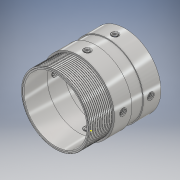
# Autodesk Inventor part: superior
Saved by Autodesk Inventor 2018 (Build 220112000, 112)
## iProperties
Created: 2019-11-08
Part Number: superior
Material: Generic
Document SubType Name: Sheet Metal
Designer: Marie
Density: 1 g/cm^3
Sheet Metal Rule: Default
Appearance: Default
Author: Marie
Autodesk Inventor part; units mm, degrees
ref_plane "XZ Plane" through (0, 0, 0) normal (0, 1, 0) x (-1, 0, 0)
ref_plane "XY Plane" through (0, 0, 0) normal (0, 0, 1) x (1, 0, 0)
sketch "Sketch1" plane through (0, 0, 0) normal (0, 0, 1) x (1, 0, 0)
  line L0 (-1.5, 60) -> (1.5, 60)
  line L1 (1.5, 60) -> (1.5, 45)
  line L2 (1.5, 45) -> (-1.5, 45)
  line L3 (-1.5, 45) -> (-1.5, 60)
  line L4 (-0.75, 45) -> (0.75, 45)
  line L5 (0.75, 45) -> (0.75, 35)
  line L6 (0.75, 35) -> (-0.75, 35)
  line L7 (-0.75, 35) -> (-0.75, 45)
  line L8 (-1.5, 35) -> (1.5, 35)
  line L9 (1.5, 35) -> (1.5, 20)
  line L10 (1.5, 20) -> (-1.5, 20)
  line L11 (-1.5, 20) -> (-1.5, 35)
  line L12 (0, 20) -> (-1.5, 20)
  line L13 (-1.5, 20) -> (-1.5, 0)
  line L14 (-1.5, 0) -> (0, 0)
  line L15 (0, 0) -> (0, 20)
  line L16 (-29.25, 61.1995) -> (-29.25, -4.0597)
  point P0 (0, 0)
  dimension "d1" = 3
  dimension "d2" = 15
  dimension "d4" = 1.5
  dimension "d5" = 10
  dimension "d8" = 3
  dimension "d9" = 15
  dimension "d10" = 1.5
  dimension "d11" = 20
  dimension "d225" = 27.75
  constraints: 34 end point, 8 parallel, 4 horizontal, 4 perpendicular, 1 midpoint, 1 point on line, 1 vertical
  measures "d1" distance of L1.end L2.end
  measures "d2" distance of L0.end L1.end
  measures "d4" distance of L5.end L6.end
  measures "d5" distance of L4.end L5.end
  measures "d8" distance of L9.end L10.end
  measures "d9" distance of L8.end L9.end
  measures "d10" distance of L14.end L13.end
  measures "d11" distance of L13.end L12.end
  measures "d225" distance between parallel lines of L13 L16
revolve "Revolution1" add sketch "Sketch1" angle 360 about axis through (-29.25, 61.1995, 0) along (0, -1, 0)
ref_plane "Work Plane2" through (1.5, 27.5, 0) normal (1, 0, 0) x (0, 1, 0)
sketch "Sketch9" plane through (1.5, 27.5, 0) normal (1, 0, 0) x (0, 1, 0)
  point P0 (-27.5, 0)
  point P1 (23.8502, 0)
  point P2 (0, 0)
hole "Hole1" at (1.5, 51.3502, 0) at (1.5, 27.5, 0) direction (-1, 0, 0) diameter 6 end through all
sketch "Sketch10" plane through (1.5, 27.5, 0) normal (1, 0, 0) x (0, 1, 0)
  point P0 (-27.5, 0)
sketch "Sketch31" plane through (-29.25, 0, 0) normal (-1, 0, 0) x (0, 0, 1)
  line L0 (29.25, 0) -> (29.25, 20)
  line L1 (29.25, 20) -> (27.0256, 20)
  line L2 (27.0256, 20) -> (27.0256, 0)
  line L3 (27.0256, 0) -> (29.25, 0)
  line L4 (0, -15.9256) -> (0, 72.6543) projected
  constraints: 8 end point
revolve "Revolution16" cut sketch "Sketch31" angle 360 about axis through (-29.25, 0, 0) along (0, 1, 0)
sketch "Sketch32" plane through (-29.25, 0, 0) normal (-1, 0, 0) x (0, 0, 1)
  line L0 (29.25, 0) -> (29.25, 20)
  line L1 (29.25, 20) -> (27.0256, 20)
  line L2 (27.0256, 20) -> (27.0256, 0)
  line L3 (27.0256, 0) -> (29.25, 0)
  line L4 (0, -15.9256) -> (0, 72.6543) projected
  constraints: 8 end point
revolve "Revolution17" add sketch "Sketch32" angle 360 about axis through (-29.25, 0, 0) along (0, 1, 0) separate body
thread "Thread13" size "M6x1" class "6H" standard "ANSI Metric M Profile" full length
thread "Thread14" size "M6x1" class "6H" standard "ANSI Metric M Profile" full length
thread "Thread15" size "M6x1" class "6H" standard "ANSI Metric M Profile" full length
thread "Thread16" size "M6x1" class "6H" standard "ANSI Metric M Profile" full length
pattern_circular "Circular Pattern2" count 4 over 360 about axis through (-29.25, 10, 0) along (0, -1, 0) of "Hole1" bodies 1
thread "Thread17" size "M6x1" class "6H" standard "ANSI Metric M Profile" full length
thread "Thread18" size "M6x1" class "6H" standard "ANSI Metric M Profile" full length
thread "Thread19" size "M6x1" class "6H" standard "ANSI Metric M Profile" full length
thread "Thread20" size "M6x1" class "6H" standard "ANSI Metric M Profile" full length
sketch "Sketch34" plane through (-56.8374, 51.3502, 0) normal (0, -1, 0) x (0, 0, 1)
  line L0 (3, 0) -> (3, 3.1626)
  line L1 (3, 3.1626) -> (2.2585, 3.1626)
  line L2 (2.2585, 3.1626) -> (2.2585, 0)
  line L3 (2.2585, 0) -> (3, 0)
  line L4 (0, -70.6399) -> (0, 15.4652) projected
  constraints: 8 end point
revolve "Revolution18" add sketch "Sketch34" angle 360 about axis through (-56.8374, 51.3502, 0) along (-1, 0, 0) separate body
sketch "Sketch33" plane through (-56.8374, 51.3502, 3) normal (0, 1, 0) x (-1, 0, 0)
  line L0 (-0.5834, -0.0507) -> (-0.5001, -0.0507) construction
  line L1 (0.0832, -0.6911) -> (-0.0001, -0.8511) construction
  line L2 (-1.0001, -0.8511) -> (-1.0834, -0.6911) construction
  line L3 (-0.4168, -0.0507) -> (-0.5001, 0.1093) construction
  line L4 (-0.5001, 0.1093) -> (-0.5834, -0.0507) construction
  line L5 (-1.0001, -0.8511) -> (-0.9168, -0.6911) construction
  line L6 (-0.4168, -0.0507) -> (-0.0834, -0.6911)
  line L7 (-1.0834, -0.6911) -> (-0.9168, -0.6911) construction
  arc A0 (-1.0834, -0.6911) -> (-1.0001, -0.7416) centre (-1.0001, -0.6477) ccw construction
  line L8 (0.0832, -0.6911) -> (-0.0834, -0.6911) construction
  line L9 (-1.0001, -0.8511) -> (-1.0001, -0.6911) construction
  line L10 (-0.0001, -0.8511) -> (-0.0001, -0.6911) construction
  line L11 (-0.5001, 0.1093) -> (-0.5001, -0.0002) construction
  line L12 (-1.0001, -0.7416) -> (-0.0001, -0.7416)
  arc A1 (-1.0001, -0.7416) -> (-0.9168, -0.6911) centre (-1.0001, -0.6477) ccw
  line L13 (-0.0834, -0.6911) -> (-0.0001, -0.8511) construction
  line L14 (-0.9168, -0.6911) -> (-0.5834, -0.0507)
  line L15 (-0.0001, -0.0002) -> (-0.0001, 0.0177)
  line L16 (-0.0001, 0.0177) -> (-0.0001, -0.0002)
  line L17 (-0.0001, -0.0002) -> (0.0334, -0.0002)
  arc A2 (-0.0834, -0.6911) -> (-0.0001, -0.7416) centre (-0.0001, -0.6477) ccw
  arc A3 (-0.0001, -0.7416) -> (0.0832, -0.6911) centre (-0.0001, -0.6477) ccw construction
  arc A4 (-0.5001, -0.0002) -> (-0.5834, -0.0507) centre (-0.5001, -0.0941) ccw
  arc A5 (-0.4168, -0.0507) -> (-0.5001, -0.0002) centre (-0.5001, -0.0941) ccw
  line L18 (-0.5001, -0.0002) -> (-0.5001, -0.0507) construction
  line L19 (-0.5001, -0.0507) -> (-0.4168, -0.0507) construction
  dimension "d289" = 55
  dimension "d290" = 0.1601
  dimension "d291" = 0.1601
  dimension "Sketch33_ThreadOffset" = 0
  dimension "Sketch33_MajorRadius" = 0.7415
  dimension "d294" = 1
  dimension "Sketch33_MinorRadius" = 0
  constraints: 40 end point, 12 point on circle, 10 parallel, 8 tangent, 6 centre point, 6 collinear, 2 midpoint, 2 point on line, 1 horizontal, 1 perpendicular, 3 other
  measures "d289" angle of L6 L14
  measures "d290" distance of L3.end L0.end
  measures "d291" distance of L1.end L10.end
  measures "Sketch33_ThreadOffset" distance between parallel lines of L15 L10
  measures "Sketch33_MajorRadius" distance from line of L12 L15.start
  measures "d294" distance from line of L1.end L9
  measures "Sketch33_MinorRadius" distance edge to line of A5 L17
coil "Coil13" sketch "Sketch33" operation cut axis through (-56.8374, 51.3502, 0) along (-1, 0, 0) pitch 1.001 turns 5.157481 hand right bodies 3
sketch "Sketch36" plane through (-56.8374, 27.5, 0) normal (0, -1, 0) x (0, 0, 1)
  line L0 (3, 0) -> (3, 3.1626)
  line L1 (3, 3.1626) -> (2.2585, 3.1626)
  line L2 (2.2585, 3.1626) -> (2.2585, 0)
  line L3 (2.2585, 0) -> (3, 0)
  line L4 (0, -70.7062) -> (0, 15.863) projected
  constraints: 8 end point
revolve "Revolution19" add sketch "Sketch36" angle 360 about axis through (-56.8374, 27.5, 0) along (-1, 0, 0) separate body
sketch "Sketch35" plane through (-56.8374, 27.5, 3) normal (0, 1, 0) x (-1, 0, 0)
  line L0 (-0.5834, -0.0507) -> (-0.5001, -0.0507) construction
  line L1 (0.0832, -0.6911) -> (-0.0001, -0.8511) construction
  line L2 (-1.0001, -0.8511) -> (-1.0834, -0.6911) construction
  line L3 (-0.4168, -0.0507) -> (-0.5001, 0.1093) construction
  line L4 (-0.5001, 0.1093) -> (-0.5834, -0.0507) construction
  line L5 (-1.0001, -0.8511) -> (-0.9168, -0.6911) construction
  line L6 (-0.4168, -0.0507) -> (-0.0834, -0.6911)
  line L7 (-1.0834, -0.6911) -> (-0.9168, -0.6911) construction
  arc A0 (-1.0834, -0.6911) -> (-1.0001, -0.7416) centre (-1.0001, -0.6477) ccw construction
  line L8 (0.0832, -0.6911) -> (-0.0834, -0.6911) construction
  line L9 (-1.0001, -0.8511) -> (-1.0001, -0.6911) construction
  line L10 (-0.0001, -0.8511) -> (-0.0001, -0.6911) construction
  line L11 (-0.5001, 0.1093) -> (-0.5001, -0.0002) construction
  line L12 (-1.0001, -0.7416) -> (-0.0001, -0.7416)
  arc A1 (-1.0001, -0.7416) -> (-0.9168, -0.6911) centre (-1.0001, -0.6477) ccw
  line L13 (-0.0834, -0.6911) -> (-0.0001, -0.8511) construction
  line L14 (-0.9168, -0.6911) -> (-0.5834, -0.0507)
  line L15 (-0.0001, -0.0002) -> (-0.0001, 0.0177)
  line L16 (-0.0001, 0.0177) -> (-0.0001, -0.0002)
  line L17 (-0.0001, -0.0002) -> (0.0334, -0.0002)
  arc A2 (-0.0834, -0.6911) -> (-0.0001, -0.7416) centre (-0.0001, -0.6477) ccw
  arc A3 (-0.0001, -0.7416) -> (0.0832, -0.6911) centre (-0.0001, -0.6477) ccw construction
  arc A4 (-0.5001, -0.0002) -> (-0.5834, -0.0507) centre (-0.5001, -0.0941) ccw
  arc A5 (-0.4168, -0.0507) -> (-0.5001, -0.0002) centre (-0.5001, -0.0941) ccw
  line L18 (-0.5001, -0.0002) -> (-0.5001, -0.0507) construction
  line L19 (-0.5001, -0.0507) -> (-0.4168, -0.0507) construction
  dimension "d307" = 55
  dimension "d308" = 0.1601
  dimension "d309" = 0.1601
  dimension "Sketch35_ThreadOffset" = 0
  dimension "Sketch35_MajorRadius" = 0.7415
  dimension "d312" = 1
  dimension "Sketch35_MinorRadius" = 0
  constraints: 40 end point, 12 point on circle, 10 parallel, 8 tangent, 6 centre point, 6 collinear, 2 midpoint, 2 point on line, 1 horizontal, 1 perpendicular, 3 other
  measures "d307" angle of L6 L14
  measures "d308" distance of L3.end L0.end
  measures "d309" distance of L1.end L10.end
  measures "Sketch35_ThreadOffset" distance between parallel lines of L15 L10
  measures "Sketch35_MajorRadius" distance from line of L12 L15.start
  measures "d312" distance from line of L1.end L9
  measures "Sketch35_MinorRadius" distance edge to line of A5 L17
coil "Coil14" sketch "Sketch35" operation cut axis through (-56.8374, 27.5, 0) along (-1, 0, 0) pitch 1.001 turns 5.157481 hand right bodies 4
sketch "Sketch38" plane through (1.5, 51.3502, 0) normal (0, -1, 0) x (0, 0, 1)
  line L0 (3, 0) -> (3, 3.1626)
  line L1 (3, 3.1626) -> (2.2585, 3.1626)
  line L2 (2.2585, 3.1626) -> (2.2585, 0)
  line L3 (2.2585, 0) -> (3, 0)
  line L4 (0, -13.6753) -> (0, 74.4181) projected
  constraints: 8 end point
revolve "Revolution20" add sketch "Sketch38" angle 360 about axis through (1.5, 51.3502, 0) along (-1, 0, 0) separate body
sketch "Sketch37" plane through (1.5, 51.3502, 3) normal (0, 1, 0) x (-1, 0, 0)
  line L0 (-0.5834, -0.0507) -> (-0.5001, -0.0507) construction
  line L1 (0.0832, -0.6911) -> (-0.0001, -0.8511) construction
  line L2 (-1.0001, -0.8511) -> (-1.0834, -0.6911) construction
  line L3 (-0.4168, -0.0507) -> (-0.5001, 0.1093) construction
  line L4 (-0.5001, 0.1093) -> (-0.5834, -0.0507) construction
  line L5 (-1.0001, -0.8511) -> (-0.9168, -0.6911) construction
  line L6 (-0.4168, -0.0507) -> (-0.0834, -0.6911)
  line L7 (-1.0834, -0.6911) -> (-0.9168, -0.6911) construction
  arc A0 (-1.0834, -0.6911) -> (-1.0001, -0.7416) centre (-1.0001, -0.6477) ccw construction
  line L8 (0.0832, -0.6911) -> (-0.0834, -0.6911) construction
  line L9 (-1.0001, -0.8511) -> (-1.0001, -0.6911) construction
  line L10 (-0.0001, -0.8511) -> (-0.0001, -0.6911) construction
  line L11 (-0.5001, 0.1093) -> (-0.5001, -0.0002) construction
  line L12 (-1.0001, -0.7416) -> (-0.0001, -0.7416)
  arc A1 (-1.0001, -0.7416) -> (-0.9168, -0.6911) centre (-1.0001, -0.6477) ccw
  line L13 (-0.0834, -0.6911) -> (-0.0001, -0.8511) construction
  line L14 (-0.9168, -0.6911) -> (-0.5834, -0.0507)
  line L15 (-0.0001, -0.0002) -> (-0.0001, 0.0177)
  line L16 (-0.0001, 0.0177) -> (-0.0001, -0.0002)
  line L17 (-0.0001, -0.0002) -> (0.0334, -0.0002)
  arc A2 (-0.0834, -0.6911) -> (-0.0001, -0.7416) centre (-0.0001, -0.6477) ccw
  arc A3 (-0.0001, -0.7416) -> (0.0832, -0.6911) centre (-0.0001, -0.6477) ccw construction
  arc A4 (-0.5001, -0.0002) -> (-0.5834, -0.0507) centre (-0.5001, -0.0941) ccw
  arc A5 (-0.4168, -0.0507) -> (-0.5001, -0.0002) centre (-0.5001, -0.0941) ccw
  line L18 (-0.5001, -0.0002) -> (-0.5001, -0.0507) construction
  line L19 (-0.5001, -0.0507) -> (-0.4168, -0.0507) construction
  dimension "d325" = 55
  dimension "d326" = 0.1601
  dimension "d327" = 0.1601
  dimension "Sketch37_ThreadOffset" = 0
  dimension "Sketch37_MajorRadius" = 0.7415
  dimension "d330" = 1
  dimension "Sketch37_MinorRadius" = 0
  constraints: 40 end point, 12 point on circle, 10 parallel, 8 tangent, 6 centre point, 6 collinear, 2 midpoint, 2 point on line, 1 horizontal, 1 perpendicular, 3 other
  measures "d325" angle of L6 L14
  measures "d326" distance of L3.end L0.end
  measures "d327" distance of L1.end L10.end
  measures "Sketch37_ThreadOffset" distance between parallel lines of L15 L10
  measures "Sketch37_MajorRadius" distance from line of L12 L15.start
  measures "d330" distance from line of L1.end L9
  measures "Sketch37_MinorRadius" distance edge to line of A5 L17
coil "Coil15" sketch "Sketch37" operation cut axis through (1.5, 51.3502, 0) along (-1, 0, 0) pitch 1.001 turns 5.157481 hand right bodies 5
sketch "Sketch40" plane through (1.5, 27.5, 0) normal (0, -1, 0) x (0, 0, 1)
  line L0 (3, 0) -> (3, 3.1626)
  line L1 (3, 3.1626) -> (2.2585, 3.1626)
  line L2 (2.2585, 3.1626) -> (2.2585, 0)
  line L3 (2.2585, 0) -> (3, 0)
  line L4 (0, -13.6753) -> (0, 74.4181) projected
  constraints: 8 end point
revolve "Revolution21" add sketch "Sketch40" angle 360 about axis through (1.5, 27.5, 0) along (-1, 0, 0) separate body
sketch "Sketch39" plane through (1.5, 27.5, 3) normal (0, 1, 0) x (-1, 0, 0)
  line L0 (-0.5834, -0.0507) -> (-0.5001, -0.0507) construction
  line L1 (0.0832, -0.6911) -> (-0.0001, -0.8511) construction
  line L2 (-1.0001, -0.8511) -> (-1.0834, -0.6911) construction
  line L3 (-0.4168, -0.0507) -> (-0.5001, 0.1093) construction
  line L4 (-0.5001, 0.1093) -> (-0.5834, -0.0507) construction
  line L5 (-1.0001, -0.8511) -> (-0.9168, -0.6911) construction
  line L6 (-0.4168, -0.0507) -> (-0.0834, -0.6911)
  line L7 (-1.0834, -0.6911) -> (-0.9168, -0.6911) construction
  arc A0 (-1.0834, -0.6911) -> (-1.0001, -0.7416) centre (-1.0001, -0.6477) ccw construction
  line L8 (0.0832, -0.6911) -> (-0.0834, -0.6911) construction
  line L9 (-1.0001, -0.8511) -> (-1.0001, -0.6911) construction
  line L10 (-0.0001, -0.8511) -> (-0.0001, -0.6911) construction
  line L11 (-0.5001, 0.1093) -> (-0.5001, -0.0002) construction
  line L12 (-1.0001, -0.7416) -> (-0.0001, -0.7416)
  arc A1 (-1.0001, -0.7416) -> (-0.9168, -0.6911) centre (-1.0001, -0.6477) ccw
  line L13 (-0.0834, -0.6911) -> (-0.0001, -0.8511) construction
  line L14 (-0.9168, -0.6911) -> (-0.5834, -0.0507)
  line L15 (-0.0001, -0.0002) -> (-0.0001, 0.0177)
  line L16 (-0.0001, 0.0177) -> (-0.0001, -0.0002)
  line L17 (-0.0001, -0.0002) -> (0.0334, -0.0002)
  arc A2 (-0.0834, -0.6911) -> (-0.0001, -0.7416) centre (-0.0001, -0.6477) ccw
  arc A3 (-0.0001, -0.7416) -> (0.0832, -0.6911) centre (-0.0001, -0.6477) ccw construction
  arc A4 (-0.5001, -0.0002) -> (-0.5834, -0.0507) centre (-0.5001, -0.0941) ccw
  arc A5 (-0.4168, -0.0507) -> (-0.5001, -0.0002) centre (-0.5001, -0.0941) ccw
  line L18 (-0.5001, -0.0002) -> (-0.5001, -0.0507) construction
  line L19 (-0.5001, -0.0507) -> (-0.4168, -0.0507) construction
  dimension "d343" = 55
  dimension "d344" = 0.1601
  dimension "d345" = 0.1601
  dimension "Sketch39_ThreadOffset" = 0
  dimension "Sketch39_MajorRadius" = 0.7415
  dimension "d348" = 1
  dimension "Sketch39_MinorRadius" = 0
  constraints: 40 end point, 12 point on circle, 10 parallel, 8 tangent, 6 centre point, 6 collinear, 2 midpoint, 2 point on line, 1 horizontal, 1 perpendicular, 3 other
  measures "d343" angle of L6 L14
  measures "d344" distance of L3.end L0.end
  measures "d345" distance of L1.end L10.end
  measures "Sketch39_ThreadOffset" distance between parallel lines of L15 L10
  measures "Sketch39_MajorRadius" distance from line of L12 L15.start
  measures "d348" distance from line of L1.end L9
  measures "Sketch39_MinorRadius" distance edge to line of A5 L17
coil "Coil16" sketch "Sketch39" operation cut axis through (1.5, 27.5, 0) along (-1, 0, 0) pitch 1.001 turns 5.157481 hand right bodies 6
sketch "Sketch42" plane through (-29.25, 51.3502, -27.5874) normal (-1, 0, 0) x (0, 1, 0)
  line L0 (3, 0) -> (3, 3.1626)
  line L1 (3, 3.1626) -> (2.2585, 3.1626)
  line L2 (2.2585, 3.1626) -> (2.2585, 0)
  line L3 (2.2585, 0) -> (3, 0)
  line L4 (0, -70.6399) -> (0, 15.4652) projected
  constraints: 8 end point
revolve "Revolution22" add sketch "Sketch42" angle 360 about axis through (-29.25, 51.3502, -27.5874) along (0, 0, -1) separate body
sketch "Sketch41" plane through (-29.25, 54.3502, -27.5874) normal (1, 0, 0) x (0, 0, -1)
  line L0 (-0.5834, -0.0507) -> (-0.5001, -0.0507) construction
  line L1 (0.0832, -0.6911) -> (-0.0001, -0.8511) construction
  line L2 (-1.0001, -0.8511) -> (-1.0834, -0.6911) construction
  line L3 (-0.4168, -0.0507) -> (-0.5001, 0.1093) construction
  line L4 (-0.5001, 0.1093) -> (-0.5834, -0.0507) construction
  line L5 (-1.0001, -0.8511) -> (-0.9168, -0.6911) construction
  line L6 (-0.4168, -0.0507) -> (-0.0834, -0.6911)
  line L7 (-1.0834, -0.6911) -> (-0.9168, -0.6911) construction
  arc A0 (-1.0834, -0.6911) -> (-1.0001, -0.7416) centre (-1.0001, -0.6477) ccw construction
  line L8 (0.0832, -0.6911) -> (-0.0834, -0.6911) construction
  line L9 (-1.0001, -0.8511) -> (-1.0001, -0.6911) construction
  line L10 (-0.0001, -0.8511) -> (-0.0001, -0.6911) construction
  line L11 (-0.5001, 0.1093) -> (-0.5001, -0.0002) construction
  line L12 (-1.0001, -0.7416) -> (-0.0001, -0.7416)
  arc A1 (-1.0001, -0.7416) -> (-0.9168, -0.6911) centre (-1.0001, -0.6477) ccw
  line L13 (-0.0834, -0.6911) -> (-0.0001, -0.8511) construction
  line L14 (-0.9168, -0.6911) -> (-0.5834, -0.0507)
  line L15 (-0.0001, -0.0002) -> (-0.0001, 0.0177)
  line L16 (-0.0001, 0.0177) -> (-0.0001, -0.0002)
  line L17 (-0.0001, -0.0002) -> (0.0334, -0.0002)
  arc A2 (-0.0834, -0.6911) -> (-0.0001, -0.7416) centre (-0.0001, -0.6477) ccw
  arc A3 (-0.0001, -0.7416) -> (0.0832, -0.6911) centre (-0.0001, -0.6477) ccw construction
  arc A4 (-0.5001, -0.0002) -> (-0.5834, -0.0507) centre (-0.5001, -0.0941) ccw
  arc A5 (-0.4168, -0.0507) -> (-0.5001, -0.0002) centre (-0.5001, -0.0941) ccw
  line L18 (-0.5001, -0.0002) -> (-0.5001, -0.0507) construction
  line L19 (-0.5001, -0.0507) -> (-0.4168, -0.0507) construction
  dimension "d361" = 55
  dimension "d362" = 0.1601
  dimension "d363" = 0.1601
  dimension "Sketch41_ThreadOffset" = 0
  dimension "Sketch41_MajorRadius" = 0.7415
  dimension "d366" = 1
  dimension "Sketch41_MinorRadius" = 0
  constraints: 40 end point, 12 point on circle, 10 parallel, 8 tangent, 6 centre point, 6 collinear, 2 midpoint, 2 point on line, 1 horizontal, 1 perpendicular, 3 other
  measures "d361" angle of L6 L14
  measures "d362" distance of L3.end L0.end
  measures "d363" distance of L1.end L10.end
  measures "Sketch41_ThreadOffset" distance between parallel lines of L15 L10
  measures "Sketch41_MajorRadius" distance from line of L12 L15.start
  measures "d366" distance from line of L1.end L9
  measures "Sketch41_MinorRadius" distance edge to line of A5 L17
coil "Coil17" sketch "Sketch41" operation cut axis through (-29.25, 51.3502, -27.5874) along (0, 0, -1) pitch 1.001 turns 5.157481 hand right bodies 7
sketch "Sketch44" plane through (-29.25, 27.5, -27.5874) normal (-1, 0, 0) x (0, 1, 0)
  line L0 (3, 0) -> (3, 3.1626)
  line L1 (3, 3.1626) -> (2.2585, 3.1626)
  line L2 (2.2585, 3.1626) -> (2.2585, 0)
  line L3 (2.2585, 0) -> (3, 0)
  line L4 (0, -70.7062) -> (0, 15.863) projected
  constraints: 8 end point
revolve "Revolution23" add sketch "Sketch44" angle 360 about axis through (-29.25, 27.5, -27.5874) along (0, 0, -1) separate body
sketch "Sketch43" plane through (-29.25, 30.5, -27.5874) normal (1, 0, 0) x (0, 0, -1)
  line L0 (-0.5834, -0.0507) -> (-0.5001, -0.0507) construction
  line L1 (0.0832, -0.6911) -> (-0.0001, -0.8511) construction
  line L2 (-1.0001, -0.8511) -> (-1.0834, -0.6911) construction
  line L3 (-0.4168, -0.0507) -> (-0.5001, 0.1093) construction
  line L4 (-0.5001, 0.1093) -> (-0.5834, -0.0507) construction
  line L5 (-1.0001, -0.8511) -> (-0.9168, -0.6911) construction
  line L6 (-0.4168, -0.0507) -> (-0.0834, -0.6911)
  line L7 (-1.0834, -0.6911) -> (-0.9168, -0.6911) construction
  arc A0 (-1.0834, -0.6911) -> (-1.0001, -0.7416) centre (-1.0001, -0.6477) ccw construction
  line L8 (0.0832, -0.6911) -> (-0.0834, -0.6911) construction
  line L9 (-1.0001, -0.8511) -> (-1.0001, -0.6911) construction
  line L10 (-0.0001, -0.8511) -> (-0.0001, -0.6911) construction
  line L11 (-0.5001, 0.1093) -> (-0.5001, -0.0002) construction
  line L12 (-1.0001, -0.7416) -> (-0.0001, -0.7416)
  arc A1 (-1.0001, -0.7416) -> (-0.9168, -0.6911) centre (-1.0001, -0.6477) ccw
  line L13 (-0.0834, -0.6911) -> (-0.0001, -0.8511) construction
  line L14 (-0.9168, -0.6911) -> (-0.5834, -0.0507)
  line L15 (-0.0001, -0.0002) -> (-0.0001, 0.0177)
  line L16 (-0.0001, 0.0177) -> (-0.0001, -0.0002)
  line L17 (-0.0001, -0.0002) -> (0.0334, -0.0002)
  arc A2 (-0.0834, -0.6911) -> (-0.0001, -0.7416) centre (-0.0001, -0.6477) ccw
  arc A3 (-0.0001, -0.7416) -> (0.0832, -0.6911) centre (-0.0001, -0.6477) ccw construction
  arc A4 (-0.5001, -0.0002) -> (-0.5834, -0.0507) centre (-0.5001, -0.0941) ccw
  arc A5 (-0.4168, -0.0507) -> (-0.5001, -0.0002) centre (-0.5001, -0.0941) ccw
  line L18 (-0.5001, -0.0002) -> (-0.5001, -0.0507) construction
  line L19 (-0.5001, -0.0507) -> (-0.4168, -0.0507) construction
  dimension "d379" = 55
  dimension "d380" = 0.1601
  dimension "d381" = 0.1601
  dimension "Sketch43_ThreadOffset" = 0
  dimension "Sketch43_MajorRadius" = 0.7415
  dimension "d384" = 1
  dimension "Sketch43_MinorRadius" = 0
  constraints: 40 end point, 12 point on circle, 10 parallel, 8 tangent, 6 centre point, 6 collinear, 2 midpoint, 2 point on line, 1 horizontal, 1 perpendicular, 3 other
  measures "d379" angle of L6 L14
  measures "d380" distance of L3.end L0.end
  measures "d381" distance of L1.end L10.end
  measures "Sketch43_ThreadOffset" distance between parallel lines of L15 L10
  measures "Sketch43_MajorRadius" distance from line of L12 L15.start
  measures "d384" distance from line of L1.end L9
  measures "Sketch43_MinorRadius" distance edge to line of A5 L17
coil "Coil18" sketch "Sketch43" operation cut axis through (-29.25, 27.5, -27.5874) along (0, 0, -1) pitch 1.001 turns 5.157481 hand right bodies 8
sketch "Sketch46" plane through (-29.25, 51.3502, 30.75) normal (-1, 0, 0) x (0, 1, 0)
  line L0 (3, 0) -> (3, 3.1626)
  line L1 (3, 3.1626) -> (2.2585, 3.1626)
  line L2 (2.2585, 3.1626) -> (2.2585, 0)
  line L3 (2.2585, 0) -> (3, 0)
  line L4 (0, -13.6753) -> (0, 74.4181) projected
  constraints: 8 end point
revolve "Revolution24" add sketch "Sketch46" angle 360 about axis through (-29.25, 51.3502, 30.75) along (0, 0, -1) separate body
sketch "Sketch45" plane through (-29.25, 54.3502, 30.75) normal (1, 0, 0) x (0, 0, -1)
  line L0 (-0.5834, -0.0507) -> (-0.5001, -0.0507) construction
  line L1 (0.0832, -0.6911) -> (-0.0001, -0.8511) construction
  line L2 (-1.0001, -0.8511) -> (-1.0834, -0.6911) construction
  line L3 (-0.4168, -0.0507) -> (-0.5001, 0.1093) construction
  line L4 (-0.5001, 0.1093) -> (-0.5834, -0.0507) construction
  line L5 (-1.0001, -0.8511) -> (-0.9168, -0.6911) construction
  line L6 (-0.4168, -0.0507) -> (-0.0834, -0.6911)
  line L7 (-1.0834, -0.6911) -> (-0.9168, -0.6911) construction
  arc A0 (-1.0834, -0.6911) -> (-1.0001, -0.7416) centre (-1.0001, -0.6477) ccw construction
  line L8 (0.0832, -0.6911) -> (-0.0834, -0.6911) construction
  line L9 (-1.0001, -0.8511) -> (-1.0001, -0.6911) construction
  line L10 (-0.0001, -0.8511) -> (-0.0001, -0.6911) construction
  line L11 (-0.5001, 0.1093) -> (-0.5001, -0.0002) construction
  line L12 (-1.0001, -0.7416) -> (-0.0001, -0.7416)
  arc A1 (-1.0001, -0.7416) -> (-0.9168, -0.6911) centre (-1.0001, -0.6477) ccw
  line L13 (-0.0834, -0.6911) -> (-0.0001, -0.8511) construction
  line L14 (-0.9168, -0.6911) -> (-0.5834, -0.0507)
  line L15 (-0.0001, -0.0002) -> (-0.0001, 0.0177)
  line L16 (-0.0001, 0.0177) -> (-0.0001, -0.0002)
  line L17 (-0.0001, -0.0002) -> (0.0334, -0.0002)
  arc A2 (-0.0834, -0.6911) -> (-0.0001, -0.7416) centre (-0.0001, -0.6477) ccw
  arc A3 (-0.0001, -0.7416) -> (0.0832, -0.6911) centre (-0.0001, -0.6477) ccw construction
  arc A4 (-0.5001, -0.0002) -> (-0.5834, -0.0507) centre (-0.5001, -0.0941) ccw
  arc A5 (-0.4168, -0.0507) -> (-0.5001, -0.0002) centre (-0.5001, -0.0941) ccw
  line L18 (-0.5001, -0.0002) -> (-0.5001, -0.0507) construction
  line L19 (-0.5001, -0.0507) -> (-0.4168, -0.0507) construction
  dimension "d397" = 55
  dimension "d398" = 0.1601
  dimension "d399" = 0.1601
  dimension "Sketch45_ThreadOffset" = 0
  dimension "Sketch45_MajorRadius" = 0.7415
  dimension "d402" = 1
  dimension "Sketch45_MinorRadius" = 0
  constraints: 40 end point, 12 point on circle, 10 parallel, 8 tangent, 6 centre point, 6 collinear, 2 midpoint, 2 point on line, 1 horizontal, 1 perpendicular, 3 other
  measures "d397" angle of L6 L14
  measures "d398" distance of L3.end L0.end
  measures "d399" distance of L1.end L10.end
  measures "Sketch45_ThreadOffset" distance between parallel lines of L15 L10
  measures "Sketch45_MajorRadius" distance from line of L12 L15.start
  measures "d402" distance from line of L1.end L9
  measures "Sketch45_MinorRadius" distance edge to line of A5 L17
coil "Coil19" sketch "Sketch45" operation cut axis through (-29.25, 51.3502, 30.75) along (0, 0, -1) pitch 1.001 turns 5.157481 hand right bodies 9
sketch "Sketch48" plane through (-29.25, 27.5, 30.75) normal (-1, 0, 0) x (0, 1, 0)
  line L0 (3, 0) -> (3, 3.1626)
  line L1 (3, 3.1626) -> (2.2585, 3.1626)
  line L2 (2.2585, 3.1626) -> (2.2585, 0)
  line L3 (2.2585, 0) -> (3, 0)
  line L4 (0, -13.6753) -> (0, 74.4181) projected
  constraints: 8 end point
revolve "Revolution25" add sketch "Sketch48" angle 360 about axis through (-29.25, 27.5, 30.75) along (0, 0, -1) separate body
sketch "Sketch47" plane through (-29.25, 30.5, 30.75) normal (1, 0, 0) x (0, 0, -1)
  line L0 (-0.5834, -0.0507) -> (-0.5001, -0.0507) construction
  line L1 (0.0832, -0.6911) -> (-0.0001, -0.8511) construction
  line L2 (-1.0001, -0.8511) -> (-1.0834, -0.6911) construction
  line L3 (-0.4168, -0.0507) -> (-0.5001, 0.1093) construction
  line L4 (-0.5001, 0.1093) -> (-0.5834, -0.0507) construction
  line L5 (-1.0001, -0.8511) -> (-0.9168, -0.6911) construction
  line L6 (-0.4168, -0.0507) -> (-0.0834, -0.6911)
  line L7 (-1.0834, -0.6911) -> (-0.9168, -0.6911) construction
  arc A0 (-1.0834, -0.6911) -> (-1.0001, -0.7416) centre (-1.0001, -0.6477) ccw construction
  line L8 (0.0832, -0.6911) -> (-0.0834, -0.6911) construction
  line L9 (-1.0001, -0.8511) -> (-1.0001, -0.6911) construction
  line L10 (-0.0001, -0.8511) -> (-0.0001, -0.6911) construction
  line L11 (-0.5001, 0.1093) -> (-0.5001, -0.0002) construction
  line L12 (-1.0001, -0.7416) -> (-0.0001, -0.7416)
  arc A1 (-1.0001, -0.7416) -> (-0.9168, -0.6911) centre (-1.0001, -0.6477) ccw
  line L13 (-0.0834, -0.6911) -> (-0.0001, -0.8511) construction
  line L14 (-0.9168, -0.6911) -> (-0.5834, -0.0507)
  line L15 (-0.0001, -0.0002) -> (-0.0001, 0.0177)
  line L16 (-0.0001, 0.0177) -> (-0.0001, -0.0002)
  line L17 (-0.0001, -0.0002) -> (0.0334, -0.0002)
  arc A2 (-0.0834, -0.6911) -> (-0.0001, -0.7416) centre (-0.0001, -0.6477) ccw
  arc A3 (-0.0001, -0.7416) -> (0.0832, -0.6911) centre (-0.0001, -0.6477) ccw construction
  arc A4 (-0.5001, -0.0002) -> (-0.5834, -0.0507) centre (-0.5001, -0.0941) ccw
  arc A5 (-0.4168, -0.0507) -> (-0.5001, -0.0002) centre (-0.5001, -0.0941) ccw
  line L18 (-0.5001, -0.0002) -> (-0.5001, -0.0507) construction
  line L19 (-0.5001, -0.0507) -> (-0.4168, -0.0507) construction
  dimension "d415" = 55
  dimension "d416" = 0.1601
  dimension "d417" = 0.1601
  dimension "Sketch47_ThreadOffset" = 0
  dimension "Sketch47_MajorRadius" = 0.7415
  dimension "d420" = 1
  dimension "Sketch47_MinorRadius" = 0
  constraints: 40 end point, 12 point on circle, 10 parallel, 8 tangent, 6 centre point, 6 collinear, 2 midpoint, 2 point on line, 1 horizontal, 1 perpendicular, 3 other
  measures "d415" angle of L6 L14
  measures "d416" distance of L3.end L0.end
  measures "d417" distance of L1.end L10.end
  measures "Sketch47_ThreadOffset" distance between parallel lines of L15 L10
  measures "Sketch47_MajorRadius" distance from line of L12 L15.start
  measures "d420" distance from line of L1.end L9
  measures "Sketch47_MinorRadius" distance edge to line of A5 L17
coil "Coil20" sketch "Sketch47" operation cut axis through (-29.25, 27.5, 30.75) along (0, 0, -1) pitch 1.001 turns 5.157481 hand right bodies 10
thread "Thread22" size "M60x1.5" class "6g" standard "ANSI Metric M Profile" full length
sketch "Sketch53" plane through (-29.25, 0, 0) normal (-1, 0, 0) x (0, 0, 1)
  line L0 (29.25, 0) -> (29.25, 20)
  line L1 (29.25, 20) -> (28.1378, 20)
  line L2 (28.1378, 20) -> (28.1378, 0)
  line L3 (28.1378, 0) -> (29.25, 0)
  line L4 (0, -13.9629) -> (0, 72.3271) projected
  constraints: 8 end point
revolve "Revolution28" cut sketch "Sketch53" angle 360 about axis through (-29.25, 0, 0) along (0, 1, 0) bodies 1
sketch "Sketch54" plane through (-29.25, 0, 0) normal (-1, 0, 0) x (0, 0, 1)
  line L0 (29.25, 0) -> (29.25, 20)
  line L1 (29.25, 20) -> (28.1378, 20)
  line L2 (28.1378, 20) -> (28.1378, 0)
  line L3 (28.1378, 0) -> (29.25, 0)
  line L4 (0, -13.9629) -> (0, 72.3271) projected
  constraints: 8 end point
revolve "Revolution29" add sketch "Sketch54" angle 360 about axis through (-29.25, 0, 0) along (0, 1, 0) separate body
sketch "Sketch52" plane through (-29.25, 0, 0) normal (1, 0, 0) x (0, 1, 0)
  line L0 (-0.8751, -28.2138) -> (-0.7501, -28.2138) construction
  line L1 (0.1249, -29.1743) -> (-0.0001, -29.4144) construction
  line L2 (-1.5001, -29.4144) -> (-1.6251, -29.1743) construction
  line L3 (-0.6251, -28.2138) -> (-0.7501, -27.9737) construction
  line L4 (-0.7501, -27.9737) -> (-0.8751, -28.2138) construction
  line L5 (-1.5001, -29.4144) -> (-1.3751, -29.1743) construction
  line L6 (-0.6251, -28.2138) -> (-0.1251, -29.1743)
  line L7 (-1.6251, -29.1743) -> (-1.3751, -29.1743) construction
  arc A0 (-1.6251, -29.1743) -> (-1.5001, -29.2502) centre (-1.5001, -29.1092) ccw construction
  line L8 (0.1249, -29.1743) -> (-0.1251, -29.1743) construction
  line L9 (-1.5001, -29.4144) -> (-1.5001, -29.1743) construction
  line L10 (-0.0001, -29.4144) -> (-0.0001, -29.1743) construction
  line L11 (-0.7501, -27.9737) -> (-0.7501, -28.138) construction
  line L12 (-1.5001, -29.2502) -> (-0.0001, -29.2502)
  arc A1 (-1.5001, -29.2502) -> (-1.3751, -29.1743) centre (-1.5001, -29.1092) ccw
  line L13 (-0.1251, -29.1743) -> (-0.0001, -29.4144) construction
  line L14 (-1.3751, -29.1743) -> (-0.8751, -28.2138)
  line L15 (-0.0001, -0.0002) -> (-0.0001, 0.0177)
  line L16 (-0.0001, 0.0177) -> (-0.0001, -0.0002)
  line L17 (-0.0001, -0.0002) -> (0.0334, -0.0002)
  arc A2 (-0.1251, -29.1743) -> (-0.0001, -29.2502) centre (-0.0001, -29.1092) ccw
  arc A3 (-0.0001, -29.2502) -> (0.1249, -29.1743) centre (-0.0001, -29.1092) ccw construction
  arc A4 (-0.7501, -28.138) -> (-0.8751, -28.2138) centre (-0.7501, -28.2789) ccw
  arc A5 (-0.6251, -28.2138) -> (-0.7501, -28.138) centre (-0.7501, -28.2789) ccw
  line L18 (-0.7501, -28.138) -> (-0.7501, -28.2138) construction
  line L19 (-0.7501, -28.2138) -> (-0.6251, -28.2138) construction
  dimension "d456" = 55
  dimension "d457" = 0.2401
  dimension "d458" = 0.2401
  dimension "Sketch52_ThreadOffset" = 0
  dimension "Sketch52_MajorRadius" = 29.25
  dimension "d461" = 1.5
  dimension "Sketch52_MinorRadius" = 28.1378
  constraints: 40 end point, 12 point on circle, 10 parallel, 8 tangent, 6 centre point, 6 collinear, 2 midpoint, 2 point on line, 1 horizontal, 1 perpendicular, 3 other
  measures "d456" angle of L6 L14
  measures "d457" distance of L3.end L0.end
  measures "d458" distance of L1.end L10.end
  measures "Sketch52_ThreadOffset" distance between parallel lines of L15 L10
  measures "Sketch52_MajorRadius" distance from line of L12 L15.start
  measures "d461" distance from line of L1.end L9
  measures "Sketch52_MinorRadius" distance edge to line of A5 L17
coil "Coil22" sketch "Sketch52" operation cut axis through (-29.25, 0, 0) along (0, 1, 0) pitch 1.5015 turns 15.318015 hand right bodies 11
equation "\"d60\" = Thickness"
equation "\"d289\" = d296"
equation "\"d290\" = 0.160083 * Sketch33_Pitch"
equation "\"d291\" = 0.160083 * Sketch33_Pitch"
equation "\"d294\" = Sketch33_Pitch"
equation "\"d307\" = d314"
equation "\"d308\" = 0.160083 * Sketch35_Pitch"
equation "\"d309\" = 0.160083 * Sketch35_Pitch"
equation "\"d312\" = Sketch35_Pitch"
equation "\"d325\" = d332"
equation "\"d326\" = 0.160083 * Sketch37_Pitch"
equation "\"d327\" = 0.160083 * Sketch37_Pitch"
equation "\"d330\" = Sketch37_Pitch"
equation "\"d343\" = d350"
equation "\"d344\" = 0.160083 * Sketch39_Pitch"
equation "\"d345\" = 0.160083 * Sketch39_Pitch"
equation "\"d348\" = Sketch39_Pitch"
equation "\"d361\" = d368"
equation "\"d362\" = 0.160083 * Sketch41_Pitch"
equation "\"d363\" = 0.160083 * Sketch41_Pitch"
equation "\"d366\" = Sketch41_Pitch"
equation "\"d379\" = d386"
equation "\"d380\" = 0.160083 * Sketch43_Pitch"
equation "\"d381\" = 0.160083 * Sketch43_Pitch"
equation "\"d384\" = Sketch43_Pitch"
equation "\"d397\" = d404"
equation "\"d398\" = 0.160083 * Sketch45_Pitch"
equation "\"d399\" = 0.160083 * Sketch45_Pitch"
equation "\"d402\" = Sketch45_Pitch"
equation "\"d415\" = d422"
equation "\"d416\" = 0.160083 * Sketch47_Pitch"
equation "\"d417\" = 0.160083 * Sketch47_Pitch"
equation "\"d420\" = Sketch47_Pitch"
equation "\"d456\" = d463"
equation "\"d457\" = 0.160083 * Sketch52_Pitch"
equation "\"d458\" = 0.160083 * Sketch52_Pitch"
equation "\"d461\" = Sketch52_Pitch"
equation "\"BendRadius\" = Thickness"
equation "\"BendReliefWidth\" = Thickness"
equation "\"BendReliefDepth\" = 0.5 * Thickness"
equation "\"CornerReliefSize\" = 4 * Thickness"
equation "\"MinimumRemnant\" = 2 * Thickness"
equation "\"TransitionRadius\" = BendRadius"
equation "\"JacobiRadiusSize\" = Thickness"
equation "\"GapSize\" = Thickness"
equation "\"d22\" = 55deg"
equation "\"Sketch2_Pitch\" = 4"
equation "\"d43\" = 55deg"
equation "\"Sketch6_Pitch\" = 4"
equation "\"d88\" = 55deg"
equation "\"Sketch11_Pitch\" = 1"
equation "\"d106\" = 55deg"
equation "\"Sketch13_Pitch\" = 1"
equation "\"d124\" = 55deg"
equation "\"Sketch15_Pitch\" = 1"
equation "\"d142\" = 55deg"
equation "\"Sketch17_Pitch\" = 1"
equation "\"d160\" = 55deg"
equation "\"Sketch19_Pitch\" = 1"
equation "\"d178\" = 55deg"
equation "\"Sketch21_Pitch\" = 1"
equation "\"d196\" = 55deg"
equation "\"Sketch23_Pitch\" = 1"
equation "\"d214\" = 55deg"
equation "\"Sketch25_Pitch\" = 1"
equation "\"d235\" = 55deg"
equation "\"Sketch27_Pitch\" = 4"
equation "\"d258\" = 55deg"
equation "\"Sketch30_Pitch\" = 3"
equation "\"d296\" = 55deg"
equation "\"Sketch33_Pitch\" = 1"
equation "\"d314\" = 55deg"
equation "\"Sketch35_Pitch\" = 1"
equation "\"d332\" = 55deg"
equation "\"Sketch37_Pitch\" = 1"
equation "\"d350\" = 55deg"
equation "\"Sketch39_Pitch\" = 1"
equation "\"d368\" = 55deg"
equation "\"Sketch41_Pitch\" = 1"
equation "\"d386\" = 55deg"
equation "\"Sketch43_Pitch\" = 1"
equation "\"d404\" = 55deg"
equation "\"Sketch45_Pitch\" = 1"
equation "\"d422\" = 55deg"
equation "\"Sketch47_Pitch\" = 1"
equation "\"d442\" = 55deg"
equation "\"Sketch49_Pitch\" = 1.5"
equation "\"d463\" = 55deg"
equation "\"Sketch52_Pitch\" = 1.5"
equation "\"Thickness\" = 0.5"
body "Solid1"
body "Solid13"
body "Solid14"
body "Solid15"
body "Solid16"
body "Solid17"
body "Solid18"
body "Solid19"
body "Solid20"
body "Solid21"
body "Solid23"
